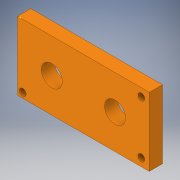
# Autodesk Inventor part: claw attachment back
Saved by Autodesk Inventor 2017 (Build 210142000, 142)
## iProperties
Created: 2018-01-10
Part Number: claw attachment back
Material: Generic
Document SubType Name: Modeling
Designer: Delta
Density: 1 g/cm^3
Appearance: Orange
Author: Delta
Autodesk Inventor part; units mm, degrees
ref_plane "YZ Plane" through (0, 0, 0) normal (1, 0, 0) x (0, 1, 0)
ref_plane "XZ Plane" through (0, 0, 0) normal (0, 1, 0) x (-1, 0, 0)
ref_plane "XY Plane" through (0, 0, 0) normal (0, 0, 1) x (1, 0, 0)
sketch "Sketch1" plane through (0, 0, 0) normal (0, 0, 1) x (1, 0, 0)
  line L0 (0, 0) -> (58.42, 0)
  line L1 (58.42, 0) -> (58.42, -33.02)
  line L2 (58.42, -33.02) -> (0, -33.02)
  line L3 (0, -33.02) -> (0, 0)
  dimension "d0" = 58.42
  dimension "d1" = 33.02
  constraints: 8 end point, 2 parallel, 1 horizontal, 1 perpendicular
  measures "d0" distance of L1.end L2.end
  measures "d1" distance of L0.end L1.end
extrude "Extrusion1" add sketch "Sketch1" along normal blind 6.35
sketch "Sketch4" plane through (0, 0, 6.35) normal (0, 0, 1) x (1, 0, 0)
  point P0 (0, 0)
sketch "Sketch5" plane through (58.42, -33.02, 0) normal (1, 0, 0) x (0, 0, -1)
  line L0 (-6.35, 33.02) -> (-6.35, 0) projected
  line L1 (0, 33.02) -> (-6.35, 33.02)
  line L2 (-6.35, 33.02) -> (-6.35, 0)
  line L3 (-6.35, 0) -> (0, 0)
  line L4 (0, 0) -> (0, 33.02)
  constraints: 8 end point, 2 parallel, 1 horizontal, 1 perpendicular
extrude "Extrusion4" add sketch "Sketch5" along normal blind 5.08
sketch "Sketch6" plane through (0, 0, 6.35) normal (0, 0, 1) x (1, 0, 0)
  circle A0 centre (15.24, -16.51) radius 5.08
  line L0 (0, 0) -> (63.5, 0) projected
  line L1 (0, 0) -> (0, -33.02) projected
  circle A1 centre (41.91, -16.51) radius 5.08
  dimension "d16" = 10.16
  dimension "d17" = 16.51
  dimension "d18" = 15.24
  dimension "d19" = 10.16
  dimension "d20" = 26.67
  constraints: 2 centre point
  measures "d16" diameter of A0
  measures "d17" distance from line of L0 A0.centre
  measures "d18" distance from line of L1 A0.centre
  measures "d19" diameter of A1
  measures "d20" distance of A1.centre A0.centre
extrude "Extrusion5" cut sketch "Sketch6" against normal blind 7.62
sketch "Sketch7" plane through (0, -33.02, 0) normal (-1, 0, 0) x (0, 0, 1)
  line L0 (6.35, 33.02) -> (6.35, 0) projected
  line L1 (0, 33.02) -> (6.35, 33.02)
  line L2 (6.35, 33.02) -> (6.35, 0)
  line L3 (6.35, 0) -> (0, 0)
  line L4 (0, 0) -> (0, 33.02)
  constraints: 8 end point, 2 parallel, 1 horizontal, 1 perpendicular
extrude "Extrusion6" add sketch "Sketch7" along normal blind 2.54
sketch "Sketch8" plane through (-2.54, -33.02, 0) normal (-1, 0, 0) x (0, 0, 1)
  line L0 (6.35, 0) -> (0, 0) projected
  line L1 (0, 33.02) -> (6.35, 33.02)
  line L2 (6.35, 33.02) -> (6.35, 0)
  line L3 (6.35, 0) -> (0, 0)
  line L4 (0, 0) -> (0, 33.02)
  constraints: 8 end point, 2 parallel, 1 horizontal, 1 perpendicular
extrude "Extrusion7" cut sketch "Sketch8" against normal blind 1.27
sketch "Sketch10" plane through (63.5, -33.02, 0) normal (1, 0, 0) x (0, 0, -1)
  line L0 (0, 33.02) -> (-6.35, 33.02) projected
  line L1 (-6.35, 33.02) -> (0, 33.02)
  line L2 (0, 33.02) -> (0, 0)
  line L3 (0, 0) -> (-6.35, 0)
  line L4 (-6.35, 0) -> (-6.35, 33.02)
  constraints: 8 end point, 2 parallel, 1 horizontal, 1 perpendicular
extrude "Extrusion9" cut sketch "Sketch10" against normal blind 1.27
sketch "Sketch11" plane through (0, 0, 6.35) normal (0, 0, 1) x (1, 0, 0)
  circle A0 centre (58.42, -3.81) radius 1.651
  circle A1 centre (58.42, -29.21) radius 1.651
  line L0 (62.23, -33.02) -> (62.23, 0) projected
  line L1 (-1.27, 0) -> (62.23, 0) projected
  line L2 (62.23, -33.02) -> (-1.27, -33.02) projected
  point P0 (0, 0)
  dimension "d37" = 3.302
  dimension "d38" = 3.302
  dimension "d39" = 3.81
  dimension "d40" = 3.81
  dimension "d41" = 3.81
  dimension "d42" = 3.81
  constraints: 2 centre point
  measures "d37" diameter of A0
  measures "d38" diameter of A1
  measures "d39" distance from line of L0 A0.centre
  measures "d40" distance from line of L1 A0.centre
  measures "d41" distance from line of A1.centre L0
  measures "d42" distance from line of A1.centre L2
extrude "Extrusion10" cut sketch "Sketch11" against normal blind 6.35
sketch "Sketch12" plane through (0, 0, 6.35) normal (0, 0, 1) x (1, 0, 0)
  circle A0 centre (1.27, -30.48) radius 1.651
  line L0 (62.23, -33.02) -> (-1.27, -33.02) projected
  line L1 (-1.27, 0) -> (-1.27, -33.02) projected
  point P0 (0, 0)
  dimension "d45" = 3.302
  dimension "d46" = 2.54
  dimension "d47" = 2.54
  constraints: 1 centre point
  measures "d45" diameter of A0
  measures "d46" distance from line of L0 A0.centre
  measures "d47" distance from line of L1 A0.centre
extrude "Extrusion11" cut sketch "Sketch12" against normal blind 6.35
sketch "Sketch14" plane through (0, 0, 6.35) normal (0, 0, 1) x (1, 0, 0)
  line L0 (62.23, -33.02) -> (-1.27, -33.02) projected
  circle A0 centre (15.24, -16.51) radius 5.08 projected
  circle A1 centre (45.72, -16.51) radius 5.08
  circle A2 centre (45.72, -16.51) radius 9.5628
  point P0 (0, 0)
  dimension "d55" = 16.51
  dimension "d56" = 30.48
  dimension "d57" = 10.16
  constraints: 2 centre point, 2 coincident
  measures "d55" distance from line of L0 point (45.72, -16.51)
  measures "d56" distance of A0.centre point (45.72, -16.51)
  measures "d57" diameter of A1
extrude "Extrusion13" add sketch "Sketch14" against normal blind 25.4 contours A2
sketch "Sketch15" plane through (0, 0, 6.35) normal (0, 0, 1) x (1, 0, 0)
  arc A0 (43.815, -21.2193) -> (43.815, -11.8007) centre (45.72, -16.51) ccw projected
  circle A1 centre (45.72, -16.51) radius 5.08
  point P0 (0, 0)
  dimension "d60" = 10.16
  constraints: 1 centre point, 1 coincident
  measures "d60" diameter of A1
extrude "Extrusion14" cut sketch "Sketch15" against normal blind 25.4
sketch "Sketch16" plane through (62.23, -33.02, 0) normal (1, 0, 0) x (0, 0, -1)
  line L0 (0, 33.02) -> (24.9561, 33.02)
  line L1 (24.9561, 33.02) -> (24.9561, -0.1066)
  line L2 (24.9561, -0.1066) -> (0, -0.1066)
  line L3 (0, -0.1066) -> (0, 33.02)
  constraints: 8 end point, 2 parallel, 1 horizontal, 1 perpendicular
extrude "Extrusion15" cut sketch "Sketch16" against normal blind 50.8
body "Solid1"
